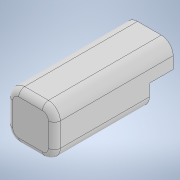
# Autodesk Inventor part: Throttle Handler
Saved by Autodesk Inventor 2020.4 (Build 244396000, 396)
## iProperties
Created: 2022-04-16
Part Number: Throttle Handler
Material: Generic
Document SubType Name: Modeling
Designer: Gurkin
Density: 1 g/cm^3
Appearance: Default
Author: Gurkin
Autodesk Inventor part; units mm, degrees
ref_plane "YZ Plane" through (0, 0, 0) normal (1, 0, 0) x (0, 1, 0)
ref_plane "XZ Plane" through (0, 0, 0) normal (0, 1, 0) x (-1, 0, 0)
ref_plane "XY Plane" through (0, 0, 0) normal (0, 0, 1) x (1, 0, 0)
sketch "Sketch1" plane through (0, 0, 0) normal (0, 0, 1) x (1, 0, 0)
  line L0 (0, 0) -> (40, 0)
  line L1 (40, 0) -> (40, 20)
  line L2 (40, 20) -> (0, 20)
  line L3 (0, 20) -> (0, 0)
  dimension "d0" = 20
  dimension "d1" = 40
  constraints: 8 end point, 2 parallel, 1 horizontal, 1 perpendicular
  measures "d0" distance between parallel lines of L0 L2
  measures "d1" distance between parallel lines of L3 L1
extrude "Extrusion1" add sketch "Sketch1" along normal blind 20
sketch "Sketch2" plane through (0, 0, 20) normal (0, 0, 1) x (1, 0, 0)
  line L0 (40, 20) -> (0, 20) projected
  line L1 (0, 20) -> (40, 20)
  line L2 (40, 20) -> (40, -20)
  line L3 (40, -20) -> (0, -20)
  line L4 (0, -20) -> (0, 20)
  point P0 (0, 0)
  dimension "d4" = 40
  dimension "d5" = 40
  constraints: 8 end point, 2 parallel, 1 horizontal, 1 perpendicular
  measures "d4" distance between parallel lines of L2 L4
  measures "d5" distance between parallel lines of L0 L3
extrude "Extrusion2" add sketch "Sketch2" along normal blind 80
fillet "Fillet1" radius 10 4 edges at (40, 20, 50) (0, 20, 50) (40, -20, 60) (0, -20, 60)
fillet "Fillet2" radius 5 8 edges at (40, 0, 100) (37.0711, -17.0711, 100) (20, -20, 100) (2.9289, -17.0711, 100) (0, 0, 100) (2.9289, 17.0711, 100) (20, 20, 100) (37.0711, 17.0711, 100)
body "Solid1"
